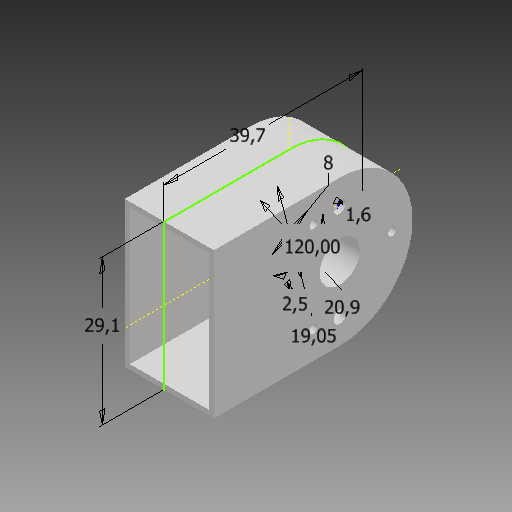
# Autodesk Inventor part: EncoderEnclosure
Saved by Autodesk Inventor 2018.3 (Build 223284000, 284)
## iProperties
Created: 2018-06-30
Part Number: EncoderEnclosure
Material: Generisch
Document SubType Name: Modeling
Designer: JochenAlt
Density: 1 g/cm^3
Appearance: Vorgabe
Author: JochenAlt
Autodesk Inventor part; units mm, degrees
ref_plane "YZ Plane" through (0, 0, 0) normal (1, 0, 0) x (0, 1, 0)
ref_plane "XZ Plane" through (0, 0, 0) normal (0, 1, 0) x (-1, 0, 0)
ref_plane "XY Plane" through (0, 0, 0) normal (0, 0, 1) x (1, 0, 0)
ref_plane "Arbeitsebene1" through (0, 0, 0) normal (1, 0, 0) x (0, 0, -1)
sketch "Skizze1" plane through (0, 0, 0) normal (1, 0, 0) x (0, 0, -1)
  arc A0 (14.55, 0) -> (-14.55, 0) centre (0, 0) ccw
  line L0 (14.55, 0) -> (14.55, -25.15)
  line L1 (14.55, -25.15) -> (-14.55, -25.15)
  line L2 (-14.55, -25.15) -> (-14.55, 0)
  circle A1 centre (0, 0) radius 4
  line L3 (-20.37, 0) -> (20.37, 0) construction
  line L4 (0, -33.09) -> (0, 22.49) construction
  circle A2 centre (0, 10.45) radius 0.8
  circle A3 centre (9.525, 0) radius 1.25
  circle A4 centre (-9.525, 0) radius 1.25
  circle A5 centre (-9.05, -5.225) radius 0.8
  circle A6 centre (9.05, -5.225) radius 0.8
  circle A7 centre (0, 0) radius 10.45 construction
  line L5 (0, 0) -> (9.05, -5.225) construction
  line L6 (0, 0) -> (-9.05, -5.225) construction
  circle A8 centre (0, 0) radius 9.525 construction
  point P0 (0, 14.55)
  dimension "d0" = 29.1
  dimension "d1" = 39.7
  dimension "d2" = 8
  dimension "d9" = 1.6
  dimension "d11" = 120
  dimension "d12" = 20.9
  dimension "d13" = 2.5
  dimension "d14" = 19.05
  constraints: 10 end point, 9 centre point, 8 point on circle, 4 coincident, 3 equal radius, 3 point on line, 1 parallel, 1 symmetric about line
  measures "d0" distance of L0.end L1.end
  measures "d1" distance from line of L1 point (0, 14.55)
  measures "d2" diameter of A1
  measures "d9" diameter of A2
  measures "d11" angle of L5 L4
  measures "d12" diameter of A7
  measures "d13" diameter of A3
  measures "d14" diameter of A8
extrude "Extrusion1" add sketch "Skizze1" along normal blind 10 and the other way blind 7.8 contours L0 L1 L2 A0 | A2 | A3 | A4 | A5 | A6
shell "Wandung1" thickness 1 removed faces 1 at (4.0667, -25.15, -4.85)
extrude "Extrusion2" cut sketch "Skizze1" against normal blind 10 from surface at 10 contours A2 | A3 | A4 | A5 | A6
